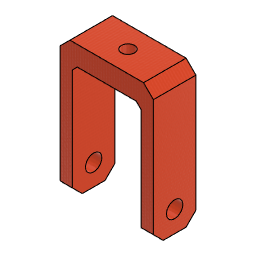
X Carrier Fork_1x (Autodesk Fusion 360 design; units mm, degrees)
Autodesk Fusion 360 part; units mm, degrees
ref_plane "WorkPlane1" through (5, -14, 2.615) normal (1, 0, 0) x (0, 1, 0)
sketch "Sketch2" plane through (5, 0, 7.615) normal (1, 0, 0) x (0, 1, 0)
  circle A0 centre (0, -31.23) radius 6.5 construction
  circle A1 centre (0, -31.23) radius 2.5
  line L0 (0, 0) -> (0, -31.23) construction
  line L1 (-6.5, 4) -> (-6.5, -31.23)
  line L2 (6.5, -31.23) -> (6.5, 4)
  line L3 (-6.5, 4) -> (6.5, 4)
  line L4 (-6.5, -2) -> (6.5, -2)
  circle A2 centre (0, 0) radius 7.615 construction
  circle A3 centre (0, -31.23) radius 7.615 construction
  line L5 (-32.934, -5.615) -> (42.066, -5.615) construction
  line L6 (42.066, -5.615) -> (42.066, -25.615) construction
  line L7 (42.066, -25.615) -> (-32.934, -25.615) construction
  line L8 (-32.934, -25.615) -> (-32.934, -5.615) construction
  line L9 (-6.5, -31.23) -> (-6.5, -37.73)
  line L10 (-6.5, -37.73) -> (6.5, -37.73)
  line L11 (6.5, -37.73) -> (6.5, -31.23)
  line L12 (6.75, 6) -> (-6.75, 6)
  dimension "d335" = 5
  dimension "d621" = 4
  dimension "d647" = 6
  dimension "d648" = 15.23
  dimension "d649" = 15.23
  dimension "d650" = 75
  dimension "d651" = 20
  dimension "d652" = 2
  dimension "d654" = 2
  dimension "d1227" = 2
  dimension "d1315" = 3.615
  dimension "d2526" = 0.25
  dimension "d3482" = 13
  constraint concentric A0 A1
  constraint coincident L0.start A2.centre
  constraint vertical L0
  constraint coincident A0.centre A1.centre
  constraint coincident A0 L1.end
  constraint tangent A0 L1
  constraint coincident A0 L2.start
  constraint tangent A0 L2
  constraint symmetric L1.start L0 L2.end
  constraint vertical L1
  constraint coincident L1.start L3.start
  constraint perpendicular L2 L3
  constraint coincident L1 L4.start
  constraint coincident L2 L4.end
  constraint perpendicular L2 L4
  constraint concentric A1 A3
  constraint horizontal L5
  constraint vertical L6
  constraint horizontal L7
  constraint vertical L8
  constraint tangent A0 L9
  constraint perpendicular L9 L10
  constraint perpendicular L10 L11
  constraint coincident L2.start L11.end
  constraint tangent A0 L10
  measures "d335" diameter of A1
  measures "d621" distance of L0.start L3
  measures "d647" distance of L2.end L4.end
  measures "d648" diameter of A2
  measures "d649" diameter of A3
  measures "d650" distance of L5.start L5.end
  measures "d651" distance of L5.start L7.end
  measures "d652" distance of A2 L5
  measures "d654" distance of A3 L7
  measures "d1227" distance of L3 L12
  measures "d1315" distance of L4.start L5
  measures "d2526" horizontal distance of L1.start L12.end
  measures "d3482" diameter of A0
extrude "Extrude3" add sketch "Sketch2" along normal blind 3.75 makes body 1
ref_plane "WorkPlane2" through (-5.5, 14, 24.515) normal (1, 0, 0) x (0, 1, 0)
chamfer "Chamfer3" distance 3 angle 45 2 edges at (6.875, 6.5, -30.115) (6.875, -6.5, -30.115) on bodies 1
mirror "Mirror2" about plane through (-5.5, 14, 24.515) normal (1, 0, 0) of bodies 1 makes body 2
extrude "Extrude5" add sketch "Sketch2" along normal blind 3.25 and the other way blind 24.25 contours L1 L2 L3 L4 bodies 1 2
sketch "Sketch3" plane through (0, 0, 5.615) normal (0, 0, -1) x (1, 0, 0)
  line L0 (-5.5, 6.5) -> (-5.5, -6.5) construction
  circle A0 centre (-5.5, 0) radius 2
  line L1 (-7.5207, -3.5) -> (-3.4793, -3.5)
  line L2 (-3.4793, -3.5) -> (-1.4585, 0)
  line L3 (-1.4585, 0) -> (-3.4793, 3.5)
  line L4 (-3.4793, 3.5) -> (-7.5207, 3.5)
  line L5 (-7.5207, 3.5) -> (-9.5415, 0)
  line L6 (-9.5415, 0) -> (-7.5207, -3.5)
  line L7 (-16, 6.5) -> (-16, -6.5)
  line L8 (-16, -6.5) -> (5, -6.5)
  line L9 (5, -6.5) -> (5, 6.5)
  line L10 (5, 6.5) -> (-16, 6.5)
  point P0 (-5.5, 0)
  dimension "d352" = 4
  dimension "d353" = 3.5
  constraint midpoint L0 P0
  constraint coincident P0 A0.centre
  constraint vertical L0
  constraint horizontal L1
  constraint midpoint L0.end L8
  constraint midpoint L0.start L10
  measures "d352" diameter of A0
  measures "d353" distance of P0 L6
extrude "Extrude6" cut sketch "Sketch3" against normal blind 19 contours A0 bodies 1
extrude "Extrude7" cut sketch "Sketch3" against normal blind 3 contours A0 | L1 L2 L3 L4 L5 L6 bodies 1
chamfer "Chamfer1" distance 1.5 angle 45 2 edges at (5, 0, 5.615) (-16, 0, 5.615) on bodies 1
chamfer "Chamfer2" distance 3 angle 45 2 edges at (8.75, 0, 11.615) (-19.75, 0, 11.615) on bodies 1
named bodies: "X Carrier Fork_1x_SN_BO"
